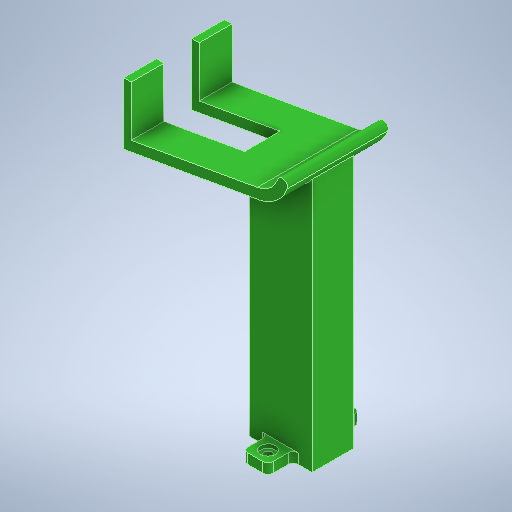
# Autodesk Inventor part: Inclined Ramp
Saved by Autodesk Inventor 2025.4 (Build 294407000, 407)
## iProperties
Created: 2026-04-06
Part Number: Inclined Ramp
Material: Generic
Document SubType Name: Modeling
Designer: lenovo
Density: 1 g/cm^3
Appearance: Default(1)
Author: lenovo
Autodesk Inventor part; units mm, degrees
ref_plane "YZ Plane" through (0, 0, 0) normal (1, 0, 0) x (0, 1, 0)
sketch "Sketch1" plane through (0, 0, 0) normal (0, 0, 1) x (1, 0, 0)
  line L0 (0, 20) -> (0, 0)
  line L1 (0, 0) -> (50, 8.8163)
  arc A0 (50, 8.8163) -> (58.1206, 15.6304) centre (48.1592, 19.256) ccw
  line L2 (0, 0) -> (58.1206, 0) construction
  line L3 (58.1206, 15.6304) -> (52.4316, 0) construction
  line L4 (0, 20) -> (-3, 20)
  line L5 (-3, 20) -> (-3, -4.5907)
  line L6 (-3, -4.5907) -> (50.6946, 4.8771)
  arc A1 (50.6946, 4.8771) -> (61.8794, 14.2623) centre (48.1592, 19.256) ccw
  arc A2 (61.8794, 14.2623) -> (58.1206, 15.6304) centre (60, 14.9463) ccw
  dimension "d1" = 20
  dimension "d2" = 50
  dimension "d3" = 3
  dimension "d4" = 70
  dimension "d5" = 2
  dimension "d6" = 10
  dimension "d7" = 10
  constraints: 14 end point, 6 point on circle, 5 tangent, 3 centre point, 2 horizontal, 1 coincident, 1 parallel, 1 perpendicular, 1 point on line, 1 vertical, 1 vertical alignment
  measures "d1" distance of L0.start L0.end
  measures "d2" horizontal distance of L0.end L1.end
  measures "d3" distance of L0.start L4.end
  measures "d4" angle of L2 L3
  measures "d5" radius of A2
  measures "d6" angle of L1 L2
  measures "d7" horizontal distance of A2.centre L1.end
extrude "Extrusion1" add sketch "Sketch1" along normal mid plane 40
sketch "Sketch2" plane through (0, 0, 0) normal (0, 1, 0) x (-1, 0, 0)
  line L0 (3, 7) -> (-32, 7)
  line L1 (-32, 7) -> (-32, -7)
  line L2 (-32, -7) -> (3, -7)
  line L3 (3, -7) -> (3, 7)
  line L4 (3, -20) -> (3, 20) projected
  point P0 (0, 0)
  point P1 (3, 0)
  point P2 (3, 0)
  dimension "d10" = 14
  dimension "d11" = 35
  constraints: 8 end point, 3 midpoint, 2 parallel, 1 coincident, 1 horizontal, 1 perpendicular
  measures "d10" distance of L2.end L0.start
  measures "d11" distance of L1.end L2.end
extrude "Extrusion2" cut sketch "Sketch2" along normal through all both and the other way through all
ref_plane "Work Plane1" through (0, -90, 0) normal (0, 1, 0) x (-1, 0, 0)
sketch "Sketch3" plane through (0, -90, 0) normal (0, 1, 0) x (-1, 0, 0)
  line L0 (-60, -8.25) -> (-35, -8.25)
  line L1 (-35, -8.25) -> (-35, 8.25)
  line L2 (-35, 8.25) -> (-60, 8.25)
  line L3 (-60, 8.25) -> (-60, -8.25)
  line L4 (-60, -8.25) -> (-35, 8.25) construction
  line L5 (-35, -8.25) -> (-60, 8.25) construction
  line L6 (-32, -7) -> (-32, 7) projected
  point P0 (0, 0)
  point P1 (-47.5, 0)
  dimension "d27" = 25
  dimension "d28" = 16.5
  dimension "d29" = 3
  constraints: 12 end point, 2 midpoint, 2 parallel, 1 horizontal, 1 horizontal alignment, 1 perpendicular
  measures "d27" distance of L2.end L1.end
  measures "d28" distance of L2.end L0.start
  measures "d29" distance between parallel lines of L6 L1
extrude "Extrusion3" add sketch "Sketch3" along normal up to next
sketch "Sketch5" plane through (42, -90, 0) normal (0, -1, 0) x (1, 0, 0)
  line L0 (15.5, 5) -> (-4.5, 5)
  line L1 (-4.5, 5) -> (-4.5, -5)
  line L2 (-4.5, -5) -> (15.5, -5)
  line L3 (15.5, -5) -> (15.5, 5)
  line L4 (15.5, 5) -> (-4.5, -5) construction
  line L5 (-4.5, 5) -> (15.5, -5) construction
  line L6 (-7, 8.25) -> (18, 8.25) projected
  line L7 (18, 8.25) -> (18, -8.25) projected
  point P0 (-42, 0)
  point P1 (5.5, 0)
  point P2 (5.5, 8.25)
  point P3 (5.5, 5)
  point P4 (18, 0)
  point P5 (15.5, 0)
  dimension "d30" = 20
  dimension "d31" = 10
  constraints: 12 end point, 6 midpoint, 2 parallel, 1 horizontal, 1 horizontal alignment, 1 perpendicular, 1 vertical alignment
  measures "d30" distance of L0.start L0.end
  measures "d31" distance between parallel lines of L0 L2
extrude "Extrusion4" cut sketch "Sketch5" against normal up to surface surface through (-3, -4.5907, 0) normal (0.1736482, -0.9848078, 0)
ref_plane "Work Plane2" through (-3, 20, 0) normal (0, 0, 1) x (1, 0, 0)
sketch "Sketch7" plane through (32, 1.5808, -7) normal (-1, 0, 0) x (0, 0, 1)
  line L0 (0, -7.9383) -> (14, -7.9383)
  line L1 (14, -7.9383) -> (14, 2.0617)
  line L2 (14, 2.0617) -> (0, 2.0617)
  line L3 (0, 2.0617) -> (0, -7.9383)
  line L4 (0, -7.9383) -> (14, 2.0617) construction
  line L5 (14, -7.9383) -> (0, 2.0617) construction
  line L6 (0, 4.0617) -> (14, 4.0617) projected
  point P0 (7, -1.5808)
  point P1 (7, -2.9383)
  point P2 (7, 4.0617)
  point P3 (7, 2.0617)
  dimension "d32" = 10
  dimension "d33" = 14
  dimension "d34" = 2
  constraints: 12 end point, 4 midpoint, 2 parallel, 1 horizontal, 1 perpendicular, 1 vertical alignment
  measures "d32" distance of L0.end L1.end
  measures "d33" distance of L1.end L2.end
  measures "d34" distance between parallel lines of L6 L2
extrude "Extrusion5" cut sketch "Sketch7" against normal up to surface (25.5 mm away)
sketch "Sketch8" plane through (35, -90, 8.25) normal (0, 0, 1) x (1, 0, 0)
  line L0 (7.5, 4) -> (17.5, 4)
  line L1 (17.5, 4) -> (17.5, 0)
  line L2 (17.5, 0) -> (7.5, 0)
  line L3 (7.5, 0) -> (7.5, 4)
  line L4 (7.5, 4) -> (17.5, 0) construction
  line L5 (17.5, 4) -> (7.5, 0) construction
  line L6 (0, 0) -> (25, 0) projected
  point P0 (-35, 90)
  point P1 (12.5, 2)
  point P2 (12.5, 0)
  point P3 (12.5, 0)
  dimension "d37" = 10
  dimension "d38" = 4
  constraints: 12 end point, 5 midpoint, 2 parallel, 1 coincident, 1 horizontal, 1 perpendicular
  measures "d37" distance of L1.end L2.end
  measures "d38" distance of L0.end L1.end
extrude "Extrusion6" add sketch "Sketch8" along normal blind 10
sketch "Sketch9" plane through (42.5, -86, 8.25) normal (0, 1, 0) x (1, 0, 0)
  circle A0 centre (5, -5) radius 1.65
  circle A1 centre (5, -5) radius 3
  line L0 (10, 0) -> (10, -10) projected
  line L1 (10, -10) -> (0, -10) projected
  point P0 (-42.5, 8.25)
  point P1 (10, -5)
  point P2 (5, -10)
  dimension "d41" = 3.3
  dimension "d42" = 6
  constraints: 2 centre point, 2 midpoint, 1 coincident, 1 horizontal alignment, 1 vertical alignment
  measures "d41" diameter of A0
  measures "d42" diameter of A1
extrude "Extrusion7" cut sketch "Sketch9" against normal through all contours A0
extrude "Extrusion8" cut sketch "Sketch9" against normal blind 1.5
fillet "Fillet1" radius 2 4 edges at (52.5, -88, 18.25) (42.5, -88, 18.25) (52.5, -88, 8.25) (42.5, -88, 8.25)
mirror "Mirror1" about plane through (0, 0, 0) normal (0, 0, 1) of "Extrusion6", "Extrusion7", "Extrusion8", "Fillet1"
fillet_without_effect "Fillet2"
body "Solid1"
